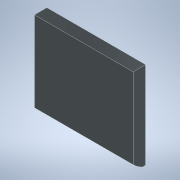
# Autodesk Inventor part: podpora silników
Saved by Autodesk Inventor 2022 (Build 260153000, 153)
## iProperties
Created: 2022-12-08
Part Number: podpora silników
Material: Lead
Document SubType Name: Modeling
Designer: Kamil
Density: 11.34 g/cm^3
Appearance: Lead
Mass: 61.3083 g
Surface Area: 29.8264 cm^2
Volume: 5.40638 cm^3
Author: Kamil
Autodesk Inventor part; units mm, degrees
ref_plane "YZ Plane" through (0, 0, 0) normal (1, 0, 0) x (0, 1, 0)
ref_plane "XZ Plane" through (0, 0, 0) normal (0, 1, 0) x (-1, 0, 0)
ref_plane "XY Plane" through (0, 0, 0) normal (0, 0, 1) x (1, 0, 0)
sketch "Sketch1" plane through (0, 0, 0) normal (0, 0, 1) x (1, 0, 0)
  line L0 (-50, 48) -> (-50, -15.8) projected
  line L1 (-50, -15.8) -> (-18.25, -15.8) projected
  line L2 (-18.25, -15.8) -> (-18.25, -48) projected
  line L3 (-18.25, -48) -> (18.25, -48) projected
  line L4 (18.25, -48) -> (18.25, -15.8) projected
  line L5 (18.25, -15.8) -> (50, -15.8) projected
  line L6 (50, -15.8) -> (50, 48) projected
  line L7 (50, 48) -> (-50, 48) projected
  line L8 (18.25, -48) -> (-18.25, -48)
  line L9 (-18.25, -48) -> (-18.25, -15.8)
  line L10 (-18.25, -15.8) -> (18.25, -15.8)
  line L11 (18.25, -15.8) -> (18.25, -48)
  point P0 (0, 0)
  constraints: 8 end point, 2 parallel, 1 horizontal, 1 perpendicular
extrude "Extrusion1" add sketch "Sketch1" along normal blind 4.6 contours L10 L4 L3 L2
sketch "Sketch2" plane through (0, 0, 4.6) normal (0, 0, 1) x (1, 0, 0)
  line L0 (-18.25, -15.8) -> (-18.25, -48) projected
  line L1 (-18.25, -48) -> (18.25, -48) projected
  line L2 (18.25, -48) -> (18.25, -15.8) projected
  line L3 (18.25, -15.8) -> (-18.25, -15.8) projected
  point P0 (0, 0)
extrude "Extrusion2" cut sketch "Sketch2" against normal blind 1
sketch "Sketch3" plane through (0, 0, 0) normal (0, 0, -1) x (-1, 0, 0)
  line L0 (4.9, -29.9) -> (18.1, -29.9)
  line L1 (4.9, -41.9) -> (18.1, -41.9)
  line L2 (-4.9, -41.9) -> (-18.1, -41.9)
  line L3 (-4.9, -29.9) -> (-18.1, -29.9)
  line L4 (11.5, -29.9) -> (11.5, -22.9)
  line L5 (-11.5, -29.9) -> (-11.5, -22.9)
  line L6 (18.25, -15.8) -> (18.25, -48) projected
  line L7 (-18.25, -15.8) -> (18.25, -15.8) projected
  line L8 (-18.25, -48) -> (-18.25, -15.8) projected
  line L9 (18.25, -48) -> (-18.25, -48) projected
  line L10 (-18.25, -15.8) -> (18.25, -15.8) projected
  line L11 (0, -15.8) -> (0, -48)
  line L12 (18.25, -48) -> (-18.25, -48) projected
  line L13 (0, -48) -> (0, -43.5)
  point P0 (0, 0)
  dimension "d4" = 7
  dimension "d5" = 4.5
  constraints: 16 end point, 4 horizontal, 4 midpoint, 3 coincident, 2 vertical, 1 point on line, 8 other
  measures "d4" distance of L4.start L4.end
  measures "d5" distance of L11.end L13.end
hole "Hole1" at (-11.5, -22.9, 0) at (11.5, -22.9, 0) direction (0, 0, 1) diameter 3 end through all
sketch "Sketch4" plane through (18.25, -48, 0) normal (1, 0, 0) x (0, 0, -1)
  arc A0 (-8.6, 4.7781) -> (-3.6, -0.73) centre (5, 12.1) ccw projected
  circle A1 centre (5, 12.1) radius 15.4457
  line L0 (-3.6, 32.2) -> (-3.6, 0) projected
  line L1 (0, 0) -> (-3.6, 0) projected
  line L2 (0, 0) -> (0, 32.2) projected
  line L3 (0, 32.2) -> (-3.6, 32.2) projected
  line L4 (0, 0) -> (0, -2.514)
  line L5 (-3.6, 0) -> (-3.6, -1.081)
  point P0 (0, 48)
  point P1 (-3.6, -0.73)
  constraints: 4 end point, 2 point on circle, 2 vertical, 1 centre point, 1 coincident
extrude "Extrusion3" add sketch "Sketch4" against normal up to surface (36.5 mm away) contours L5 L1 L4 A1
body "Solid1"
